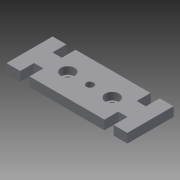
# Autodesk Inventor part: prepazka-sablona
Saved by Autodesk Inventor 2015 (Build 190159000, 159)
## iProperties
Created: 2012-08-25
Part Number: prepazka-sablona
Material: Generic
Document SubType Name: Modeling
Designer: idle-rug
Density: 1 g/cm^3
Appearance: Default
Author: idle-rug
Autodesk Inventor part; units mm, degrees
ref_plane "YZ Plane" through (0, 0, 0) normal (1, 0, 0) x (0, 1, 0)
ref_plane "XZ Plane" through (0, 0, 0) normal (0, 1, 0) x (-1, 0, 0)
ref_plane "XY Plane" through (0, 0, 0) normal (0, 0, 1) x (1, 0, 0)
sketch "Sketch1" plane through (0, 0, 0) normal (0, 0, 1) x (1, 0, 0)
  line L0 (65.5, 25) -> (-65.5, 25)
  line L1 (-65.5, 25) -> (-65.5, -25)
  line L2 (-65.5, -25) -> (65.5, -25)
  line L3 (65.5, -25) -> (65.5, 25)
  line L4 (-40.6, 25) -> (-40.6, 10)
  line L5 (-40.6, 10) -> (-50.6, 10)
  line L6 (-50.6, 10) -> (-50.6, 25)
  line L7 (-40.6, -25) -> (-40.6, -10)
  line L8 (-40.6, -10) -> (-50.6, -10)
  line L9 (-50.6, -10) -> (-50.6, -25)
  line L10 (40.6, 25) -> (40.6, 10)
  line L11 (40.6, 10) -> (50.6, 10)
  line L12 (50.6, 10) -> (50.6, 25)
  line L13 (40.6, -25) -> (40.6, -10)
  line L14 (40.6, -10) -> (50.6, -10)
  line L15 (50.6, -10) -> (50.6, -25)
  circle A0 centre (24.1, 0) radius 7.5
  circle A1 centre (-24.1, 0) radius 7.5
  circle A2 centre (24.1, 0) radius 7.5
  circle A3 centre (-24.1, 0) radius 7.5
  circle A4 centre (0, 0) radius 4
  dimension "d0" = 15
  dimension "d1" = 15
  dimension "d2" = 15
  dimension "d3" = 15
  dimension "d8" = 15
  dimension "d9" = 15
  dimension "d30" = 8
  constraints: 32 end point, 8 point on line, 7 perpendicular, 5 centre point, 2 concentric, 1 coincident
  measures "d0" distance of L4.start L4.end
  measures "d1" distance of L7.start L7.end
  measures "d2" distance of L10.start L10.end
  measures "d3" distance of L13.start L13.end
  measures "d8" diameter of A0
  measures "d9" diameter of A1
  measures "d30" diameter of A4
extrude "Extrusion2" add sketch "Sketch1" along normal blind 10 contours L3 L2 L15 L14 L13 L7 L8 L9 L1 L0 L6 L5 L4 L10 L11 L12 | A4
sketch "Sketch2" plane through (-40.6, 25, 0) normal (0, 1, 0) x (1, 0, 0)
  circle A0 centre (64.7, -5) radius 1.25
  circle A1 centre (16.5, -5) radius 1.25
  point P0 (40.6, 0)
  dimension "d15" = 2.5
  dimension "d16" = 2.5
  constraints: 2 centre point
  measures "d15" diameter of A0
  measures "d16" diameter of A1
extrude "Extrusion3" cut sketch "Sketch2" against normal blind 10
sketch "Sketch3" plane through (0, 0, 0) normal (0, 0, -1) x (-1, 0, 0)
  circle A0 centre (0, 0) radius 24.1
  circle A1 centre (-24.1, 0) radius 5
  circle A2 centre (24.1, 0) radius 5
  circle A3 centre (-24.1, 0) radius 7.5
  circle A4 centre (24.1, 0) radius 7.5
  dimension "d25" = 48.2
  dimension "d26" = 10
  dimension "d27" = 10
  constraints: 5 centre point, 3 coincident, 2 point on circle
  measures "d25" diameter of A0
  measures "d26" diameter of A1
  measures "d27" diameter of A2
extrude "Extrusion6" add sketch "Sketch3" against normal blind 2 contours A2 A0 A4 | A0 A4 A2 | A3 A0 A1 | A0 A1 A3
extrude "Extrusion7" cut sketch "Sketch1" along normal blind 10 contours A4
body "Solid2"
